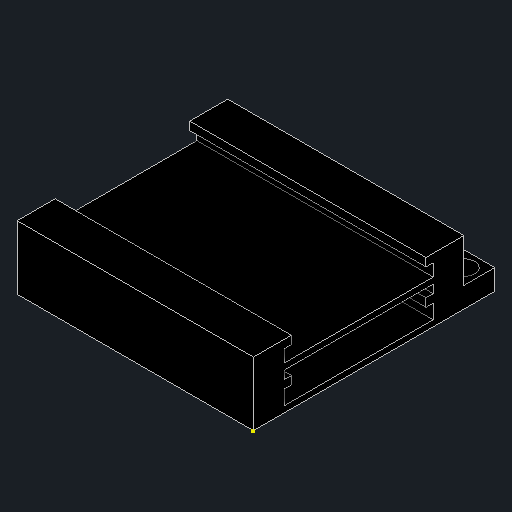
# Autodesk Inventor part: drvholder
Saved by Autodesk Inventor 2026.2 (Build 302298010, 298A)
## iProperties
Created: 2026-05-10
Part Number: drvholder
Material: Tworzywo sztuczne PET
Document SubType Name: Modeling
Designer: karol
Density: 1.541 g/cm^3
Appearance: Poliwęglan — przezroczysty
Author: karol
Autodesk Inventor part; units mm, degrees
ref_plane "YZ Plane" through (0, 0, 0) normal (1, 0, 0) x (0, 1, 0)
ref_plane "XZ Plane" through (0, 0, 0) normal (0, 1, 0) x (-1, 0, 0)
ref_plane "XY Plane" through (0, 0, 0) normal (0, 0, 1) x (1, 0, 0)
sketch "Sketch1" plane through (0, 0, 0) normal (0, 1, 0) x (-1, 0, 0)
  line L0 (0, 0) -> (23, 0)
  line L1 (23, 0) -> (23, -3)
  line L2 (23, -3) -> (0, -3)
  line L3 (0, -3) -> (0, 0)
  line L4 (23, -3) -> (0, -3)
  line L5 (0, -3) -> (0, -17.5)
  line L6 (0, -17.5) -> (23, -17.5)
  line L7 (23, -17.5) -> (23, -3)
  line L8 (23, -17.5) -> (0, -17.5)
  line L9 (0, -17.5) -> (0, -20.5)
  line L10 (0, -20.5) -> (23, -20.5)
  line L11 (23, -20.5) -> (23, -17.5)
  dimension "d0" = 23
  dimension "d1" = 3
  dimension "d2" = 14.5
  dimension "d3" = 3
  constraints: 24 end point, 6 parallel, 3 horizontal, 3 perpendicular, 2 point on line
  measures "d0" distance of L1.end L2.end
  measures "d1" distance of L0.end L1.end
  measures "d2" distance of L5.end L4.end
  measures "d3" distance of L9.end L8.end
extrude "Extrusion1" add sketch "Sketch1" along normal blind 5 contours L0 L1 L2 L3 | L6 L11 L10 L9
sketch "Sketch2" plane through (0, 0, -3) normal (0, 0, -1) x (-1, 0, 0)
  line L0 (0, 0) -> (0, 5) projected
  line L1 (23, 0) -> (23, 5) projected
  line L2 (0, 1.8) -> (23, 1.8)
  line L3 (23, 1.8) -> (23, 1)
  line L4 (23, 1) -> (0, 1)
  line L5 (0, 1) -> (0, 1.8)
  line L6 (0, 0) -> (23, 0) projected
  point P0 (0, 1)
  dimension "d6" = 0.8
  dimension "d7" = 1
  constraints: 8 end point, 2 parallel, 2 point on line, 1 horizontal, 1 perpendicular
  measures "d6" distance of L2.end L3.end
  measures "d7" distance between parallel lines of L6 L4
extrude "Extrusion2" add sketch "Sketch2" along normal up to surface (14.5 mm away) contours L0 L2 L1 L4
sketch "Sketch3" plane through (-23, 5, -17.5) normal (0, 0, 1) x (1, 0, 0)
  line L0 (0, -5) -> (0, 0) projected
  line L1 (23, -5) -> (23, 0) projected
  line L2 (0, -1.9) -> (23, -1.9)
  line L3 (23, -1.9) -> (23, -2.7)
  line L4 (23, -2.7) -> (0, -2.7)
  line L5 (0, -2.7) -> (0, -1.9)
  line L6 (0, -3.2) -> (23, -3.2) projected
  point P0 (0, -2.7)
  dimension "d10" = 0.8
  dimension "d11" = 0.5
  constraints: 8 end point, 2 parallel, 2 point on line, 1 horizontal, 1 perpendicular
  measures "d10" distance of L2.end L3.end
  measures "d11" distance between parallel lines of L6 L4
extrude "Extrusion3" add sketch "Sketch3" along normal blind 0.7 contours L0 L2 L1 L4
sketch "Sketch4" plane through (0, 5, -3) normal (0, 0, -1) x (-1, 0, 0)
  line L0 (0, -2.7) -> (0, -1.9) projected
  line L1 (0, -1.9) -> (23, -1.9) projected
  line L2 (23, -1.9) -> (23, -2.7) projected
  line L3 (23, -2.7) -> (0, -2.7) projected
  point P0 (0, -5)
extrude "Extrusion4" add sketch "Sketch4" along normal blind 0.7
sketch "Sketch5" plane through (0, 5, 0) normal (0, 1, 0) x (1, 0, 0)
  line L0 (-23, 0) -> (0, 0) projected
  line L1 (0, 0) -> (0, 3) projected
  line L2 (0, 3) -> (-23, 3) projected
  line L3 (-23, 3) -> (-23, 0) projected
  line L4 (-23, 17.5) -> (0, 17.5) projected
  line L5 (0, 17.5) -> (0, 20.5) projected
  line L6 (0, 20.5) -> (-23, 20.5) projected
  line L7 (-23, 20.5) -> (-23, 17.5) projected
extrude "Extrusion5" add sketch "Sketch5" along normal blind 1.5
sketch "Sketch6" plane through (0, 3.1, -3) normal (0, 0, -1) x (-1, 0, 0)
  line L0 (0, 3.4) -> (23, 3.4) projected
  line L1 (23, 0) -> (23, 3.4) projected
  line L2 (0, 3.4) -> (23, 3.4)
  line L3 (23, 3.4) -> (23, 2.6)
  line L4 (23, 2.6) -> (0, 2.6)
  line L5 (0, 2.6) -> (0, 3.4)
  point P0 (0, -3.1)
  dimension "d18" = 0.8
  constraints: 8 end point, 2 parallel, 1 horizontal, 1 perpendicular, 1 point on line
  measures "d18" distance of L2.end L3.end
extrude "Extrusion6" add sketch "Sketch6" along normal blind 0.7
sketch "Sketch7" plane through (-23, 3.1, -17.5) normal (0, 0, 1) x (1, 0, 0)
  line L0 (23, 2.6) -> (0, 2.6) projected
  line L1 (0, 2.6) -> (0, 3.4) projected
  line L2 (0, 3.4) -> (23, 3.4) projected
  line L3 (23, 3.4) -> (23, 2.6) projected
  point P0 (23, -3.1)
extrude "Extrusion7" add sketch "Sketch7" along normal blind 0.7
sketch "Sketch8" plane through (-23, 3.1, -17.5) normal (0, 0, 1) x (1, 0, 0)
  line L0 (23, 0) -> (23, 2.6) projected
  line L1 (0, 0) -> (0, 2.6) projected
  line L2 (23, 2.1) -> (0, 2.1)
  line L3 (0, 2.1) -> (0, 1.3)
  line L4 (0, 1.3) -> (23, 1.3)
  line L5 (23, 1.3) -> (23, 2.1)
  line L6 (23, 3.4) -> (0, 3.4) projected
  point P0 (23, -3.1)
  point P1 (0, 2.1)
  dimension "d23" = 0.8
  dimension "d24" = 1.3
  constraints: 8 end point, 2 parallel, 1 horizontal, 1 midpoint, 1 perpendicular, 1 point on line
  measures "d23" distance of L3.end L2.end
  measures "d24" distance between parallel lines of L6 L2
extrude "Extrusion8" add sketch "Sketch8" along normal up to surface (14.5 mm away)
sketch "Sketch9" plane through (0, 0, 0) normal (0, -1, 0) x (1, 0, 0)
  line L0 (-23, -17.5) -> (0, -17.5) projected
  line L1 (-23, -20.5) -> (-23, -17.5) projected
  line L2 (0, -20.5) -> (-23, -20.5) projected
  line L3 (0, -17.5) -> (0, -20.5) projected
  line L4 (-23, 0) -> (0, 0) projected
  line L5 (-23, -3) -> (-23, 0) projected
  line L6 (0, -3) -> (-23, -3) projected
  line L7 (0, 0) -> (0, -3) projected
extrude "Extrusion9" cut sketch "Sketch9" against normal blind 0.3
sketch "Sketch10" plane through (0, 6.5, -20.5) normal (0, 0, -1) x (-1, 0, 0)
  line L0 (23, -6.2) -> (0, -6.2) projected
  line L1 (0, -6.2) -> (3, -6.2)
  line L2 (3, -6.2) -> (3, -4.2)
  line L3 (3, -4.2) -> (0, -4.2)
  line L4 (0, -4.2) -> (0, -6.2)
  point P0 (0, -6.5)
  dimension "d29" = 3
  dimension "d30" = 2
  constraints: 8 end point, 2 parallel, 1 horizontal, 1 perpendicular
  measures "d29" distance of L3.end L2.end
  measures "d30" distance of L2.end L1.end
extrude "Extrusion10" add sketch "Sketch10" along normal blind 3
sketch "Sketch11" plane through (0, 6.5, -20.5) normal (0, 0, -1) x (-1, 0, 0)
  line L0 (23, -6.2) -> (0, -6.2) projected
  line L1 (23, -6.2) -> (20, -6.2)
  line L2 (20, -6.2) -> (20, -4.2)
  line L3 (20, -4.2) -> (23, -4.2)
  line L4 (23, -4.2) -> (23, -6.2)
  point P0 (0, -6.5)
  dimension "d33" = 3
  dimension "d34" = 2
  constraints: 8 end point, 2 parallel, 1 horizontal, 1 perpendicular
  measures "d33" distance of L2.end L3.end
  measures "d34" distance of L1.end L2.end
extrude "Extrusion11" add sketch "Sketch11" along normal blind 3
sketch "Sketch12" plane through (-3, 2.3, -20.5) normal (0, 1, 0) x (1, 0, 0)
  circle A0 centre (1.5, 1.5) radius 1.05
  line L0 (3, 0) -> (3, 3) projected
  line L1 (0, 3) -> (3, 3) projected
  circle A1 centre (-18.5, 1.5) radius 1.05
  line L2 (-17, 0) -> (-17, 3) projected
  line L3 (-20, 3) -> (-17, 3) projected
  point P0 (3, -20.5)
  point P1 (1.5, 3)
  point P2 (-17, 1.5)
  point P3 (-18.5, 3)
  dimension "d37" = 2.1
  dimension "d38" = 1.5
  dimension "d39" = 1.5
  dimension "d40" = 2.1
  dimension "d41" = 1.5
  dimension "d42" = 1.5
  constraints: 3 midpoint, 2 centre point
  measures "d37" diameter of A0
  measures "d38" distance from line of L0 A0.centre
  measures "d39" distance of point (1.5, 3) A0.centre
  measures "d40" diameter of A1
  measures "d41" distance of point (-17, 1.5) A1.centre
  measures "d42" distance of point (-18.5, 3) A1.centre
extrude "Extrusion12" cut sketch "Sketch12" against normal blind 2
sketch "Sketch13" plane through (-20, 0.3, -20.5) normal (1, 0, 0) x (0, 0, -1)
  line L0 (-3, 4.1) -> (-17.5, 4.1) projected
  line L1 (-3, 2.8) -> (-3, 4.1) projected
  line L2 (-3, 2.8) -> (-3.7, 2.8) projected
  line L3 (-3.7, 2) -> (-3.7, 2.8) projected
  line L4 (-3, 2) -> (-3.7, 2) projected
  line L5 (-3, 1.5) -> (-3, 2) projected
  line L6 (-17.5, 1.5) -> (-3, 1.5) projected
  line L7 (-17.5, 1.5) -> (-17.5, 2) projected
  line L8 (-17.5, 2) -> (-16.8, 2) projected
  line L9 (-16.8, 2.8) -> (-16.8, 2) projected
  line L10 (-17.5, 2.8) -> (-16.8, 2.8) projected
  line L11 (-17.5, 2.8) -> (-17.5, 4.1) projected
  line L12 (-20.5, 0) -> (-17.5, 0) projected
  line L13 (-17.5, 0) -> (-17.5, 0.7) projected
  line L14 (-17.5, 0.7) -> (-3, 0.7) projected
  line L15 (-3, 0) -> (-3, 0.7) projected
  line L16 (-3, 0) -> (3, 0) projected
  line L17 (3, 2) -> (3, 0) projected
  line L18 (0, 2) -> (3, 2) projected
  line L19 (0, 2) -> (0, 6.2) projected
  line L20 (0, 6.2) -> (-3.7, 6.2) projected
  line L21 (-3.7, 5.4) -> (-3.7, 6.2) projected
  line L22 (-3, 5.4) -> (-3.7, 5.4) projected
  line L23 (-3, 4.9) -> (-3, 5.4) projected
  line L24 (-3, 4.9) -> (-17.5, 4.9) projected
  line L25 (-17.5, 4.9) -> (-17.5, 5.4) projected
  line L26 (-17.5, 5.4) -> (-16.8, 5.4) projected
  line L27 (-16.8, 6.2) -> (-16.8, 5.4) projected
  line L28 (-20.5, 6.2) -> (-16.8, 6.2) projected
  line L29 (-20.5, 0) -> (-20.5, 6.2) projected
  line L30 (0, 0) -> (0, 2) projected
  line L31 (0, 0) -> (3, 0) projected
  line L32 (3, 2) -> (3, 0) projected
  line L33 (0, 2) -> (3, 2) projected
  point P0 (-20.5, -0.3)
extrude "Extrusion13" add sketch "Sketch13" along normal up to surface (17 mm away) contours L30 L18 L17 L16
sketch "Sketch14" plane through (-23, 1, -3) normal (0, -1, 0) x (1, 0, 0)
  line L0 (23, -14.5) -> (0, -14.5) projected
  line L1 (23, 0) -> (23, -14.5) projected
  line L2 (0, 0) -> (23, 0) projected
  line L3 (0, 0) -> (0, -14.5) projected
  point P0 (23, 3)
extrude "Extrusion14" cut sketch "Sketch14" against normal blind 0.8
sketch "Sketch15" plane through (0, 0.3, 0) normal (0, -1, 0) x (1, 0, 0)
  point P0 (0, 0)
sketch "Sketch16" plane through (0, 0.3, 0) normal (0, -1, 0) x (1, 0, 0)
  circle A0 centre (-21.5, -22) radius 1.05 projected
  circle A1 centre (-1.5, -22) radius 1.05 projected
  line L0 (0, -17.5) -> (0, -23.5) projected
  line L1 (-23, -17.5) -> (0, -17.5) projected
  line L2 (-23, -23.5) -> (-23, -17.5) projected
  line L3 (0, -23.5) -> (-23, -23.5) projected
  line L4 (-23, -3) -> (0, -3) projected
  line L5 (-23, -17.5) -> (-23, -3) projected
  line L6 (0, -17.5) -> (-23, -17.5) projected
  line L7 (0, -17.5) -> (0, -3) projected
  point P0 (0, 0)
extrude "Extrusion15" add sketch "Sketch16" against normal blind 0.6 contours L1 L5 L4 L7
sketch "Sketch17" plane through (-23, 4.4, -17.5) normal (0, -1, 0) x (1, 0, 0)
  line L0 (0, 14.5) -> (23, 14.5) projected
  line L1 (0, 0) -> (0, 14.5) projected
  line L2 (23, 0) -> (0, 0) projected
  line L3 (23, 0) -> (23, 14.5) projected
  point P0 (23, 17.5)
extrude "Extrusion16" add sketch "Sketch17" along normal blind 0.5
sketch "Sketch18" plane through (-23, 5.2, -17.5) normal (0, 1, 0) x (1, 0, 0)
  line L0 (23, -14.5) -> (0, -14.5) projected
  line L1 (23, 0) -> (23, -14.5) projected
  line L2 (0, 0) -> (23, 0) projected
  line L3 (0, 0) -> (0, -14.5) projected
  point P0 (23, -17.5)
extrude "Extrusion17" cut sketch "Sketch18" against normal blind 0.7
body "Solid1"
